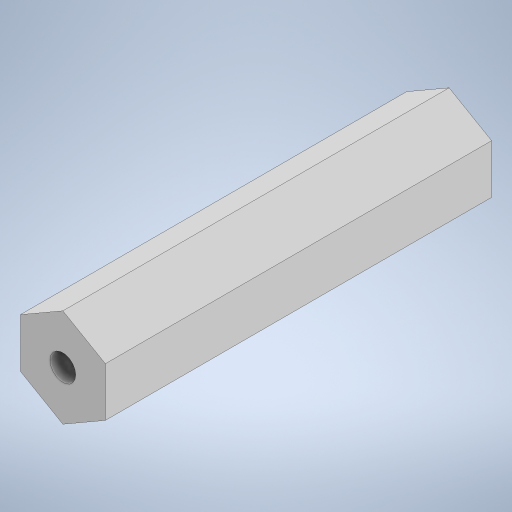
# Autodesk Inventor part: Standoff_V1
Saved by Autodesk Inventor 2024 (Build 280153000, 153)
## iProperties
Created: 2024-06-06
Part Number: Standoff_V1
Material: Generic
Document SubType Name: Modeling
Designer: Hemant
Density: 1 g/cm^3
Appearance: Default
Author: Hemant
Autodesk Inventor part; units mm, degrees
ref_plane "YZ Plane" through (0, 0, 0) normal (1, 0, 0) x (0, 1, 0)
ref_plane "XZ Plane" through (0, 0, 0) normal (0, 1, 0) x (-1, 0, 0)
ref_plane "XY Plane" through (0, 0, 0) normal (0, 0, 1) x (1, 0, 0)
sketch "Sketch1" plane through (0, 0, 0) normal (0, 0, 1) x (1, 0, 0)
  circle A0 centre (0, 0) radius 0.9 construction
  circle A1 centre (0, 0) radius 3.3 construction
  line L0 (3.3, -1.9053) -> (0, -3.8105)
  line L1 (0, -3.8105) -> (-3.3, -1.9053)
  line L2 (-3.3, -1.9053) -> (-3.3, 1.9053)
  line L3 (-3.3, 1.9053) -> (0, 3.8105)
  line L4 (0, 3.8105) -> (3.3, 1.9053)
  line L5 (3.3, 1.9053) -> (3.3, -1.9053)
  circle A2 centre (0, 0) radius 0.6
  point P0 (3.3, 0)
  dimension "d0" = 1.8
  dimension "d1" = 2.4
  dimension "d4" = 1.2
  constraints: 12 end point, 3 coincident, 2 centre point, 1 horizontal alignment, 1 midpoint, 15 other
  measures "d0" diameter of A0
  measures "d4" diameter of A2
extrude "Extrusion1" add sketch "Sketch1" along normal blind 30
sketch "Sketch2" plane through (0, 0, 0) normal (0, 0, -1) x (-1, 0, 0)
  circle A0 centre (0, 0) radius 0.6 projected
  constraints: 1 coincident
hole "Hole1" at (0, 0, 0) direction (0, 0, 1) diameter 2 end through all
body "Solid1"
